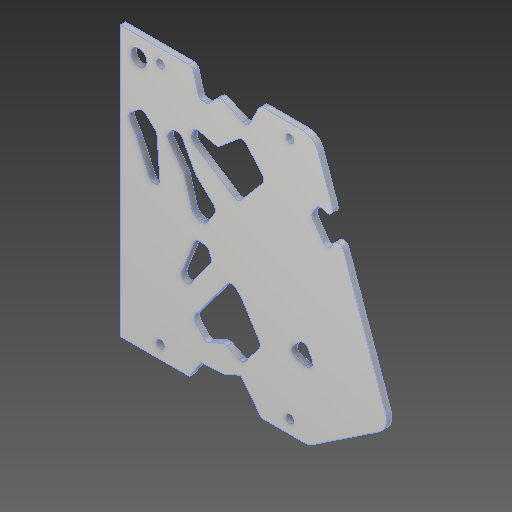
# Autodesk Inventor part: palmrest-plate
Saved by Autodesk Inventor 2018 (Build 220112000, 112)
## iProperties
Created: 2018-07-10
Part Number: palmrest-plate
Material: アルミニウム 6061
Document SubType Name: Sheet Metal
Designer: NaMACHAN
Mass: 37.9044 g
Surface Area: 156.062 cm^2
Volume: 14.0387 cm^3
Density: 2.7 g/cm^3
Sheet Metal Rule: Default
Appearance: アルミニウム - フラット
Author: NaMACHAN
Autodesk Inventor part; units mm, degrees
ref_plane "YZ Plane" through (0, 0, 0) normal (1, 0, 0) x (0, 1, 0)
ref_plane "XZ Plane" through (0, 0, 0) normal (0, 1, 0) x (-1, 0, 0)
ref_plane "XY Plane" through (0, 0, 0) normal (0, 0, 1) x (1, 0, 0)
ref_plane "作業平面1" through (0, 0, 0) normal (0, 0, 1) x (1, 0, 0)
sketch "スケッチ1" plane through (0, 0, 0) normal (0, 0, 1) x (1, 0, 0)
  line L0 (38, 50) -> (34, 50)
  line L1 (-34, 50) -> (34, 50)
  line L2 (38, 50) -> (38, -50)
  line L3 (-38, -50) -> (-38, 50)
  circle A0 centre (-19, -45) radius 1.5
  circle A1 centre (-19, 45) radius 1.5
  circle A2 centre (29, 45) radius 1.5
  circle A3 centre (29, -45) radius 1.5
  circle A4 centre (-27, 43) radius 3
  line L4 (38, 50) -> (66, -30)
  line L5 (66, -30) -> (36, -50)
  line L6 (36, -50) -> (-34, -50)
  line L7 (-34, -50) -> (-34, 50)
  point P0 (0, 0)
  dimension "d0" = 70
  dimension "d1" = 30
  dimension "d2" = 20
  measures "d0" distance of L5.end L6.end
  measures "d1" horizontal distance of L5.end L4.end
  measures "d2" vertical distance of L4.end L5.end
extrude "プレート1" add sketch "スケッチ1" along normal blind 2
fillet "コーナーR1" radius 6 3 edges at (66, -30, 1) (36, -50, 1) (38, 50, 1)
sketch "スケッチ2" plane through (0, 0, 2) normal (0, 0, 1) x (1, 0, 0)
  line L0 (-11.9603, -25.5927) -> (0.1995, -8.9635)
  line L1 (0.1995, -8.9635) -> (-1.3072, -5.066)
  line L2 (-1.3072, -5.066) -> (-5.8804, -4.5176)
  line L3 (-5.8804, -4.5176) -> (-13.8957, -24.8289)
  line L4 (-13.8957, -24.8289) -> (-11.9603, -25.5927)
  line L5 (9.7633, 14.8381) -> (19.9789, 26.8894)
  line L6 (19.9789, 26.8894) -> (11.5513, 36.8214)
  line L7 (11.5513, 36.8214) -> (2.2529, 28.9314)
  line L8 (2.2529, 28.9314) -> (-6.5978, 31.0395)
  line L9 (-6.5978, 31.0395) -> (-7.7328, 26.2742)
  line L10 (-7.7328, 26.2742) -> (9.7633, 14.8381)
  line L11 (-2.1719, 1.9898) -> (2.0176, 8.3993)
  line L12 (2.0176, 8.3993) -> (-5.8804, 15.9409)
  line L13 (-5.8804, 15.9409) -> (-11.395, 26.2742)
  line L14 (-11.395, 26.2742) -> (-14.5226, 26.2742)
  line L15 (-34, -50) -> (-34, 50) projected
  line L16 (-14.5226, 26.2742) -> (-16.8005, 23.1589)
  line L17 (-16.8005, 23.1589) -> (-10.2186, 14.1226)
  line L18 (-10.2186, 14.1226) -> (-7.1653, 3.4592)
  line L19 (-7.1653, 3.4592) -> (-4.9173, 1.9898)
  line L20 (-4.9173, 1.9898) -> (-2.1719, 1.9898)
  line L21 (-20.3606, 0.7763) -> (-27.7925, 16.9418)
  line L22 (-27.7925, 16.9418) -> (-31.3415, 22.8283)
  line L23 (-31.3415, 22.8283) -> (-25.8511, 27.4871)
  line L24 (-25.8511, 27.4871) -> (-20.3606, 22.2701)
  line L25 (-20.3606, 22.2701) -> (-18.852, 2.4818)
  line L26 (-18.852, 2.4818) -> (-20.3606, 0.7763)
  line L27 (-7.1653, -30.3189) -> (7.1386, -11.3918)
  line L28 (7.1386, -11.3918) -> (10.9777, -14.9782)
  line L29 (10.9777, -14.9782) -> (18.5067, -26.9403)
  line L30 (18.5067, -26.9403) -> (11.5513, -36.1438)
  line L31 (11.5513, -36.1438) -> (4.7809, -32.8107)
  line L32 (4.7809, -32.8107) -> (-2.1719, -36.1438)
  line L33 (-2.1719, -36.1438) -> (-7.1653, -30.3189)
  line L34 (34.1833, -50) -> (-34, -50) projected
  line L35 (-8.3134, -50) -> (-3.9925, -43.3895)
  line L36 (-3.9925, -43.3895) -> (5.251, -42.7096)
  line L37 (5.251, -42.7096) -> (10.6786, -40.1077)
  line L38 (10.6786, -40.1077) -> (18.5067, -50)
  line L39 (-8.3134, -50) -> (18.5067, -50)
  line L40 (27.8184, -23.5083) -> (35.8003, -25.3016)
  line L41 (35.8003, -25.3016) -> (38.1252, -23.3085)
  line L42 (38.1252, -23.3085) -> (34.2868, -16.5841)
  line L43 (34.2868, -16.5841) -> (27.8184, -23.5083)
  line L44 (43.2555, 14.8879) -> (36.7435, 24.4627)
  line L45 (36.7435, 24.4627) -> (39.7583, 29.4784)
  line L46 (39.7583, 29.4784) -> (46.6277, 25.3494)
  line L47 (39.4063, 45.9821) -> (64.4625, -25.6072) projected
  line L48 (43.2555, 14.8879) -> (47.0439, 24.1602)
  line L49 (46.6277, 25.3494) -> (47.0439, 24.1602)
  line L50 (-34, 50) -> (33.7431, 50) projected
  line L51 (17.8703, 50) -> (13.3521, 40.8223)
  line L52 (13.3521, 40.8223) -> (2.9186, 45.4111)
  line L53 (2.9186, 45.4111) -> (-1.4965, 40.8223)
  line L54 (-1.4965, 40.8223) -> (-4.6686, 40.8223)
  line L55 (-4.6686, 40.8223) -> (-7.1653, 50)
  line L56 (-7.1653, 50) -> (17.8703, 50)
  point P0 (0, 0)
  constraints: 106 end point, 7 perpendicular, 7 point on line, 5 parallel, 2 collinear
extrude "押し出し1" cut sketch "スケッチ2" against normal blind 10
fillet "コーナーR2" radius 2 48 edges at (4.7809, -32.8107, 1) (11.5513, -36.1438, 1) (-2.1719, -36.1438, 1) (-7.1653, -30.3189, 1) (7.1386, -11.3918, 1) (10.9777, -14.9782, 1) (18.5067, -26.9403, 1) (27.8184, -23.5083, 1) (35.8003, -25.3016, 1) (38.1252, -23.3085, 1) (34.2868, -16.5841, 1) (43.2555, 14.8879, 1) (47.0439, 24.1602, 1) (46.6277, 25.3494, 1) (39.7583, 29.4784, 1) (36.7435, 24.4627, 1) (17.8703, 50, 1) (13.3521, 40.8223, 1) (2.9186, 45.4111, 1) (-1.4965, 40.8223, 1) (-4.6686, 40.8223, 1) (-7.1653, 50, 1) (2.2529, 28.9314, 1) (11.5513, 36.8214, 1) (19.9789, 26.8894, 1) (9.7633, 14.8381, 1) (-7.7328, 26.2742, 1) (-6.5978, 31.0395, 1) (-14.5226, 26.2742, 1) (-11.395, 26.2742, 1) (-5.8804, 15.9409, 1) (2.0176, 8.3993, 1) (-2.1719, 1.9898, 1) (-4.9173, 1.9898, 1) (-7.1653, 3.4592, 1) (-10.2186, 14.1226, 1) (-16.8005, 23.1589, 1) (-20.3606, 22.2701, 1) (-25.8511, 27.4871, 1) (-31.3415, 22.8283, 1) (-27.7925, 16.9418, 1) (-18.852, 2.4818, 1) (-20.3606, 0.7763, 1) (-5.8804, -4.5176, 1) (-1.3072, -5.066, 1) (0.1995, -8.9635, 1) (-11.9603, -25.5927, 1) (-13.8957, -24.8289, 1)
equation "\"d3\" = Thickness"
equation "\"BendRadius\" = Thickness"
equation "\"BendReliefWidth\" = Thickness"
equation "\"BendReliefDepth\" = 0.5 * Thickness"
equation "\"CornerReliefSize\" = 4 * Thickness"
equation "\"MinimumRemnant\" = 2 * Thickness"
equation "\"TransitionRadius\" = BendRadius"
equation "\"JacobiRadiusSize\" = Thickness"
equation "\"GapSize\" = Thickness"
equation "\"Thickness\" = 2"
